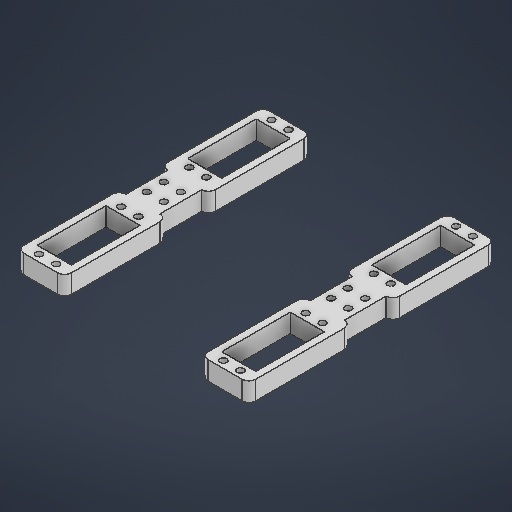
# Autodesk Inventor part: robot_7_chassis
Saved by Autodesk Inventor 2026.1 (Build 301233000, 233)
## iProperties
Created: 2026-05-05
Part Number: robot_7_chassis
Material: Generic
Document SubType Name: Modeling
Designer: emanuel
Density: 1 g/cm^3
Appearance: Default
Author: emanuel
Autodesk Inventor part; units mm, degrees
ref_plane "YZ Plane" through (0, 0, 0) normal (1, 0, 0) x (0, 1, 0)
ref_plane "XZ Plane" through (0, 0, 0) normal (0, 1, 0) x (-1, 0, 0)
ref_plane "XY Plane" through (0, 0, 0) normal (0, 0, 1) x (1, 0, 0)
sketch "Sketch1" plane through (0, 0, 0) normal (0, 1, 0) x (-1, 0, 0)
  line L0 (0, 0) -> (54.15, 0)
  line L1 (54.15, 20) -> (54.15, -20)
  line L2 (49.15, -20) -> (59.15, -20)
  circle A0 centre (59.15, -20) radius 2
  circle A1 centre (49.15, -20) radius 2
  line L3 (59.15, -20) -> (49.15, -20)
  line L4 (49.15, -20) -> (49.15, -68.3)
  line L5 (49.15, -68.3) -> (59.15, -68.3)
  line L6 (59.15, -68.3) -> (59.15, -20)
  circle A2 centre (59.15, -68.3) radius 2
  circle A3 centre (49.15, -68.3) radius 2
  line L7 (59.15, -20) -> (64.15, -20)
  line L8 (64.15, -20) -> (64.15, -16)
  line L9 (64.15, -16) -> (59.15, -16)
  line L10 (59.15, -16) -> (59.15, -20)
  line L11 (49.15, -20) -> (44.15, -20)
  line L12 (44.15, -20) -> (44.15, -24)
  line L13 (44.15, -24) -> (49.15, -24)
  line L14 (49.15, -24) -> (49.15, -20)
  line L15 (64.15, -16) -> (44.15, -16)
  line L16 (44.15, -16) -> (44.15, -24)
  line L17 (44.15, -24) -> (64.15, -24)
  line L18 (64.15, -24) -> (64.15, -16)
  line L19 (59.15, -68.3) -> (64.15, -68.3)
  line L20 (64.15, -68.3) -> (64.15, -72.3)
  line L21 (64.15, -72.3) -> (59.15, -72.3)
  line L22 (59.15, -72.3) -> (59.15, -68.3)
  line L23 (49.15, -68.3) -> (44.15, -68.3)
  line L24 (44.15, -68.3) -> (44.15, -64.3)
  line L25 (44.15, -64.3) -> (49.15, -64.3)
  line L26 (49.15, -64.3) -> (49.15, -68.3)
  line L27 (44.15, -64.3) -> (64.15, -64.3)
  line L28 (64.15, -64.3) -> (64.15, -72.3)
  line L29 (64.15, -72.3) -> (44.15, -72.3)
  line L30 (44.15, -72.3) -> (44.15, -64.3)
  line L31 (54.15, -20) -> (54.15, -68.3)
  line L32 (54.15, -20) -> (54.15, 20)
  line L33 (49.15, 20) -> (59.15, 20)
  circle A4 centre (59.15, 20) radius 2
  circle A5 centre (49.15, 20) radius 2
  line L34 (59.15, 20) -> (49.15, 20)
  line L35 (49.15, 20) -> (49.15, 68.3)
  line L36 (49.15, 68.3) -> (59.15, 68.3)
  line L37 (59.15, 68.3) -> (59.15, 20)
  circle A6 centre (59.15, 68.3) radius 2
  circle A7 centre (49.15, 68.3) radius 2
  line L38 (59.15, 20) -> (64.15, 20)
  line L39 (64.15, 20) -> (64.15, 16)
  line L40 (64.15, 16) -> (59.15, 16)
  line L41 (59.15, 16) -> (59.15, 20)
  line L42 (49.15, 20) -> (44.15, 20)
  line L43 (44.15, 20) -> (44.15, 24)
  line L44 (44.15, 24) -> (49.15, 24)
  line L45 (49.15, 24) -> (49.15, 20)
  line L46 (64.15, 16) -> (44.15, 16)
  line L47 (44.15, 16) -> (44.15, 24)
  line L48 (44.15, 24) -> (64.15, 24)
  line L49 (64.15, 24) -> (64.15, 16)
  line L50 (59.15, 68.3) -> (64.15, 68.3)
  line L51 (64.15, 68.3) -> (64.15, 72.3)
  line L52 (64.15, 72.3) -> (59.15, 72.3)
  line L53 (59.15, 72.3) -> (59.15, 68.3)
  line L54 (49.15, 68.3) -> (44.15, 68.3)
  line L55 (44.15, 68.3) -> (44.15, 64.3)
  line L56 (44.15, 64.3) -> (49.15, 64.3)
  line L57 (49.15, 64.3) -> (49.15, 68.3)
  line L58 (44.15, 64.3) -> (64.15, 64.3)
  line L59 (64.15, 64.3) -> (64.15, 72.3)
  line L60 (64.15, 72.3) -> (44.15, 72.3)
  line L61 (44.15, 72.3) -> (44.15, 64.3)
  line L62 (54.15, 20) -> (54.15, 68.3)
  line L63 (0, 5) -> (0, -5)
  line L64 (0, 0) -> (-54.15, 0)
  line L65 (-54.15, 20) -> (-54.15, -20)
  line L66 (-49.15, -20) -> (-59.15, -20)
  circle A8 centre (-59.15, -20) radius 2
  circle A9 centre (-49.15, -20) radius 2
  line L67 (-59.15, -20) -> (-49.15, -20)
  line L68 (-49.15, -20) -> (-49.15, -68.3)
  line L69 (-49.15, -68.3) -> (-59.15, -68.3)
  line L70 (-59.15, -68.3) -> (-59.15, -20)
  circle A10 centre (-59.15, -68.3) radius 2
  circle A11 centre (-49.15, -68.3) radius 2
  line L71 (-59.15, -20) -> (-64.15, -20)
  line L72 (-64.15, -20) -> (-64.15, -16)
  line L73 (-64.15, -16) -> (-59.15, -16)
  line L74 (-59.15, -16) -> (-59.15, -20)
  line L75 (-49.15, -20) -> (-44.15, -20)
  line L76 (-44.15, -20) -> (-44.15, -24)
  line L77 (-44.15, -24) -> (-49.15, -24)
  line L78 (-49.15, -24) -> (-49.15, -20)
  line L79 (-64.15, -16) -> (-44.15, -16)
  line L80 (-44.15, -16) -> (-44.15, -24)
  line L81 (-44.15, -24) -> (-64.15, -24)
  line L82 (-64.15, -24) -> (-64.15, -16)
  line L83 (-59.15, -68.3) -> (-64.15, -68.3)
  line L84 (-64.15, -68.3) -> (-64.15, -72.3)
  line L85 (-64.15, -72.3) -> (-59.15, -72.3)
  line L86 (-59.15, -72.3) -> (-59.15, -68.3)
  line L87 (-49.15, -68.3) -> (-44.15, -68.3)
  line L88 (-44.15, -68.3) -> (-44.15, -64.3)
  line L89 (-44.15, -64.3) -> (-49.15, -64.3)
  line L90 (-49.15, -64.3) -> (-49.15, -68.3)
  line L91 (-44.15, -64.3) -> (-64.15, -64.3)
  line L92 (-64.15, -64.3) -> (-64.15, -72.3)
  line L93 (-64.15, -72.3) -> (-44.15, -72.3)
  line L94 (-44.15, -72.3) -> (-44.15, -64.3)
  line L95 (-54.15, -20) -> (-54.15, -68.3)
  circle A12 centre (-59.15, 20) radius 2
  line L96 (-64.15, 16) -> (-44.15, 16)
  line L97 (-44.15, 16) -> (-44.15, 24)
  circle A13 centre (-49.15, 20) radius 2
  line L98 (-49.15, 20) -> (-59.15, 20)
  line L99 (-59.15, 20) -> (-49.15, 20)
  line L100 (-44.15, 24) -> (-64.15, 24)
  line L101 (-44.15, 24) -> (-49.15, 24)
  line L102 (-44.15, 20) -> (-44.15, 24)
  line L103 (-59.15, 68.3) -> (-59.15, 20)
  line L104 (-54.15, 20) -> (-54.15, 68.3)
  line L105 (-49.15, 20) -> (-49.15, 68.3)
  line L106 (-49.15, 24) -> (-49.15, 20)
  line L107 (-59.15, 20) -> (-64.15, 20)
  line L108 (-59.15, 16) -> (-59.15, 20)
  line L109 (-64.15, 24) -> (-64.15, 16)
  line L110 (-64.15, 20) -> (-64.15, 16)
  line L111 (-64.15, 16) -> (-59.15, 16)
  line L112 (-49.15, 68.3) -> (-59.15, 68.3)
  circle A14 centre (-59.15, 68.3) radius 2
  circle A15 centre (-49.15, 68.3) radius 2
  line L113 (-44.15, 64.3) -> (-49.15, 64.3)
  line L114 (-44.15, 64.3) -> (-64.15, 64.3)
  line L115 (-44.15, 68.3) -> (-44.15, 64.3)
  line L116 (-49.15, 64.3) -> (-49.15, 68.3)
  line L117 (-59.15, 68.3) -> (-64.15, 68.3)
  line L118 (-44.15, 72.3) -> (-44.15, 64.3)
  line L119 (-59.15, 72.3) -> (-59.15, 68.3)
  line L120 (-64.15, 64.3) -> (-64.15, 72.3)
  line L121 (-64.15, 68.3) -> (-64.15, 72.3)
  line L122 (-64.15, 72.3) -> (-59.15, 72.3)
  line L123 (-64.15, 72.3) -> (-44.15, 72.3)
  line L124 (-49.15, 68.3) -> (-44.15, 68.3)
  line L125 (-49.15, 20) -> (-44.15, 20)
  line L126 (-54.15, -20) -> (-54.15, 20)
  point P0 (64.15, -20)
  point P1 (-49.15, 24)
  point P2 (-64.15, 20)
  dimension "d0" = 54.15
  dimension "d1" = 40
  dimension "d3" = 10
  dimension "d6" = 4
  dimension "d7" = 4
  dimension "d11" = 48.3
  dimension "d12" = 4
  dimension "d13" = 4
  dimension "d14" = 5
  dimension "d15" = 4
  dimension "d16" = 5
  dimension "d17" = 4
  dimension "d18" = 5
  dimension "d19" = 4
  dimension "d20" = 5
  dimension "d21" = 4
  dimension "d22" = 10
  constraints: 254 end point, 85 symmetric about line, 16 centre point, 16 coincident, 14 parallel, 8 horizontal, 7 perpendicular, 4 midpoint, 2 vertical, 12 other
  measures "d0" distance of L0.start L0.end
  measures "d1" distance of L1.start L1.end
  measures "d3" distance of L2.start L2.end
  measures "d6" diameter of A0
  measures "d7" diameter of A1
  measures "d11" distance of L4.end L3.end
  measures "d12" diameter of A2
  measures "d13" diameter of A3
  measures "d14" distance of L9.end L8.end
  measures "d15" distance of L8.end L7.end
  measures "d16" distance of L13.end L12.end
  measures "d17" distance of L12.end L11.end
  measures "d18" distance of L20.end L21.end
  measures "d19" distance of L19.end L20.end
  measures "d20" distance of L24.end L25.end
  measures "d21" distance of L23.end L24.end
  measures "d22" distance of L63.start L63.end
extrude "Extrusion1" add sketch "Sketch1" along normal blind 11 contours L46 L47 L42 A5 L33 L1 | L1 L33 A4 L41 L46 | L15 L10 A0 L2 L1 | L1 L2 A1 L11 L16 L15 | L79 L80 L75 A9 L66 L65 | L65 L66 A8 L74 L79 | L96 L108 A12 L98 L65 | L65 L98 A13 L125 L97 L96 | L62 L48 L37 A4 L33 | L33 A5 L35 L48 L62 | L41 A4 L38 L39 L40 | L31 L17 L4 A1 L2 | L2 A0 L6 L17 L31 | L9 L8 L7 A0 L10 | L104 L100 L105 A13 L98 | L98 A12 L103 L100 L104 | L96 L109 L107 A12 L108 | L95 L81 L70 A8 L66 | L66 A9 L68 L81 L95 | L74 A8 L71 L72 L73 | L43 L44 L35 A5 L42 | L11 A1 L4 L13 L12 | L125 A13 L105 L100 L97 | L76 L77 L68 A9 L75 | L37 L48 L49 L38 A4 | L62 L36 A6 L37 L58 | L58 L35 A7 L36 L62 | A0 L7 L18 L17 L6 | L31 L5 A3 L4 L27 | L27 L6 A2 L5 L31 | A12 L107 L109 L100 L103 | L114 L103 A14 L112 L104 | L104 L112 A15 L105 L114 | L70 L81 L82 L71 A8 | L95 L69 A10 L70 L91 | L91 L68 A11 L69 L95 | L56 L55 L54 A7 L35 | L37 A6 L50 L59 L58 | L36 A7 L54 L61 L60 L53 A6 | L4 A3 L23 L24 L25 | L27 L28 L19 A2 L6 | L5 A2 L22 L29 L30 L23 A3 | L105 A15 L124 L115 L113 | L114 L120 L117 A14 L103 | L112 A14 L119 L123 L118 L124 A15 | L89 L88 L87 A11 L68 | L70 A10 L83 L92 L91 | L69 A11 L87 L94 L93 L86 A10 | A6 L53 L52 L51 L50 | L19 L20 L21 L22 A2 | L117 L120 L122 L119 A14 | A10 L86 L85 L84 L83
sketch "Sketch4" plane through (0, 11, 0) normal (0, 1, 0) x (1, 0, 0)
  line L0 (64.15, 64.3) -> (64.15, 72.3) projected
  line L1 (64.15, 72.3) -> (68.15, 72.3)
  line L2 (68.15, 72.3) -> (68.15, 12.3)
  line L3 (68.15, 12.3) -> (64.15, 12.3)
  line L4 (64.15, 12.3) -> (64.15, 72.3)
  line L5 (44.15, 72.3) -> (44.15, 64.3) projected
  line L6 (44.15, 72.3) -> (40.15, 72.3)
  line L7 (40.15, 72.3) -> (40.15, 12.3)
  line L8 (40.15, 12.3) -> (44.15, 12.3)
  line L9 (44.15, 12.3) -> (44.15, 72.3)
  line L10 (-44.15, 64.3) -> (-44.15, 72.3) projected
  line L11 (-44.15, 72.3) -> (-40.15, 72.3)
  line L12 (-40.15, 72.3) -> (-40.15, 12.3)
  line L13 (-40.15, 12.3) -> (-44.15, 12.3)
  line L14 (-44.15, 12.3) -> (-44.15, 72.3)
  line L15 (-64.15, 72.3) -> (-64.15, 64.3) projected
  line L16 (-64.15, 72.3) -> (-68.15, 72.3)
  line L17 (-68.15, 72.3) -> (-68.15, 12.3)
  line L18 (-68.15, 12.3) -> (-64.15, 12.3)
  line L19 (-64.15, 12.3) -> (-64.15, 72.3)
  line L20 (-64.15, -72.3) -> (-44.15, -72.3) projected
  line L21 (-44.15, -72.3) -> (-40.15, -72.3)
  line L22 (-40.15, -72.3) -> (-40.15, -12.3)
  line L23 (-40.15, -12.3) -> (-44.15, -12.3)
  line L24 (-44.15, -12.3) -> (-44.15, -72.3)
  line L25 (44.15, -72.3) -> (40.15, -72.3)
  line L26 (40.15, -72.3) -> (40.15, -12.3)
  line L27 (40.15, -12.3) -> (44.15, -12.3)
  line L28 (44.15, -12.3) -> (44.15, -72.3)
  line L29 (64.15, -72.3) -> (68.15, -72.3)
  line L30 (68.15, -72.3) -> (68.15, -12.3)
  line L31 (68.15, -12.3) -> (64.15, -12.3)
  line L32 (64.15, -12.3) -> (64.15, -72.3)
  line L33 (-64.15, -72.3) -> (-68.15, -72.3)
  line L34 (-68.15, -72.3) -> (-68.15, -12.3)
  line L35 (-68.15, -12.3) -> (-64.15, -12.3)
  line L36 (-64.15, -12.3) -> (-64.15, -72.3)
  point P0 (0, 0)
  dimension "d35" = 4
  dimension "d36" = 60
  dimension "d37" = 4
  dimension "d38" = 60
  dimension "d39" = 4
  dimension "d40" = 60
  dimension "d41" = 4
  dimension "d42" = 60
  dimension "d43" = 4
  dimension "d44" = 60
  constraints: 64 end point, 16 parallel, 10 point on line, 8 horizontal, 8 perpendicular
  measures "d35" distance of L2.end L3.end
  measures "d36" distance of L1.end L2.end
  measures "d37" distance of L8.end L7.end
  measures "d38" distance of L7.end L6.end
  measures "d39" distance of L12.end L13.end
  measures "d40" distance of L11.end L12.end
  measures "d41" distance of L18.end L17.end
  measures "d42" distance of L17.end L16.end
  measures "d43" distance of L23.end L22.end
  measures "d44" distance of L22.end L21.end
extrude "Extrusion4" add sketch "Sketch4" against normal up to surface (11 mm away)
fillet "Fillet1" radius 4 16 edges at (-40.15, 5.5, 12.3) (-40.15, 5.5, -12.3) (40.15, 5.5, 12.3) (40.15, 5.5, -12.3) (68.15, 5.5, 12.3) (68.15, 5.5, -12.3) (-68.15, 5.5, 12.3) (-68.15, 5.5, -12.3) (-68.15, 5.5, 72.3) (68.15, 5.5, 72.3) (68.15, 5.5, -72.3) (-68.15, 5.5, -72.3) (-40.15, 5.5, 72.3) (-40.15, 5.5, -72.3) (40.15, 5.5, -72.3) (40.15, 5.5, 72.3)
sketch "Sketch5" plane through (0, 11, 0) normal (0, 1, 0) x (1, 0, 0)
  arc A0 (-68.15, 16.3) -> (-64.15, 12.3) centre (-64.15, 16.3) ccw projected
  line L0 (-44.15, -16) -> (-64.15, -16) projected
  line L1 (-64.15, 16.3) -> (-44.15, 16.3)
  line L2 (-44.15, 16.3) -> (-44.15, -16)
  line L3 (-44.15, -16) -> (-64.15, -16)
  line L4 (-64.15, -16) -> (-64.15, 16.3)
  line L5 (44.15, 12.3) -> (44.15, 16) projected
  line L6 (64.15, -16) -> (64.15, -12.3) projected
  line L7 (44.15, 16) -> (64.15, 16)
  line L8 (64.15, 16) -> (64.15, -16)
  line L9 (64.15, -16) -> (44.15, -16)
  line L10 (44.15, -16) -> (44.15, 16)
  line L11 (-54.15, 16.3) -> (-54.15, 0)
  line L12 (-59.15, -5) -> (-49.15, -5)
  line L13 (-49.15, -5) -> (-49.15, 5)
  line L14 (-49.15, 5) -> (-59.15, 5)
  line L15 (-59.15, 5) -> (-59.15, -5)
  line L16 (-59.15, -5) -> (-49.15, 5) construction
  line L17 (-49.15, -5) -> (-59.15, 5) construction
  circle A1 centre (-59.15, 5) radius 2
  circle A2 centre (-49.15, 5) radius 2
  circle A3 centre (-59.15, -5) radius 2
  circle A4 centre (-49.15, -5) radius 2
  line L18 (54.15, 16) -> (54.15, 0)
  line L19 (49.15, -5) -> (59.15, -5)
  line L20 (59.15, -5) -> (59.15, 5)
  line L21 (59.15, 5) -> (49.15, 5)
  line L22 (49.15, 5) -> (49.15, -5)
  line L23 (49.15, -5) -> (59.15, 5) construction
  line L24 (59.15, -5) -> (49.15, 5) construction
  circle A5 centre (48.9333, 5) radius 2
  circle A6 centre (59.15, 5) radius 2
  circle A7 centre (49.15, -5) radius 2
  circle A8 centre (59.15, -5) radius 2
  point P0 (0, 0)
  dimension "d48" = 10
  dimension "d49" = 10
  dimension "d50" = 4
  dimension "d51" = 4
  dimension "d52" = 4
  dimension "d53" = 4
  dimension "d54" = 10
  dimension "d55" = 10
  dimension "d56" = 4
  dimension "d57" = 4
  dimension "d58" = 4
  dimension "d59" = 4
  constraints: 44 end point, 8 centre point, 8 parallel, 7 coincident, 6 midpoint, 5 perpendicular, 4 horizontal, 1 vertical
  measures "d48" distance of L14.end L13.end
  measures "d49" distance of L13.end L12.end
  measures "d50" diameter of A1
  measures "d51" diameter of A2
  measures "d52" diameter of A3
  measures "d53" diameter of A4
  measures "d54" distance of L21.end L20.end
  measures "d55" distance of L20.end L19.end
  measures "d56" diameter of A5
  measures "d57" diameter of A6
  measures "d58" diameter of A7
  measures "d59" diameter of A8
extrude "Extrusion5" add sketch "Sketch5" against normal up to surface (11 mm away) contours L14 A2 L13 A4 L12 A3 L15 A1 | L0 L4 L1 L2 | L21 A6 L20 A8 L19 A7 L22 A5 | L5 L7 L8 L6 L9 L10
body "Solid1"
